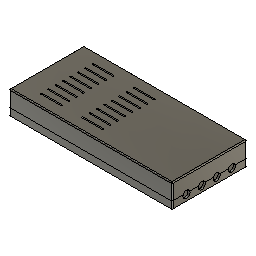
bladeRF_micro_b200_case (Autodesk Fusion 360 design; units mm, degrees)
Autodesk Fusion 360 part; units mm, degrees
(part 1 of 14)
sketch "micro (1)" plane through (0, 0, 0) normal (0, 0, 1) x (1, 0, 0)
  line L0 (35.86, 33.621) -> (35.86, 34.221)
  line L1 (35.86, 34.221) -> (34.76, 34.221)
  line L2 (34.76, 34.221) -> (34.76, 33.621)
  line L3 (41.36, 56.942) -> (41.36, 56.342)
  line L4 (35.818, 34.2258) -> (35.818, 33.6162)
  line L5 (42.46, 59.228) -> (41.36, 59.228)
  line L6 (42.418, 59.2328) -> (42.418, 58.6232)
  line L7 (42.46, 56.942) -> (41.36, 56.942)
  line L8 (35.818, 34.2258) -> (35.818, 33.6162)
  line L9 (42.035, 56.3372) -> (42.035, 56.9468)
  line L10 (41.36, 56.342) -> (42.46, 56.342)
  line L11 (29.591, 15.3162) -> (28.575, 15.3162)
  line L12 (41.785, 58.6232) -> (42.035, 58.6232)
  line L13 (41.785, 56.3372) -> (42.035, 56.3372)
  line L14 (41.402, 56.9468) -> (42.418, 56.9468)
  line L15 (41.402, 58.6232) -> (41.402, 59.2328)
  line L16 (42.035, 58.6232) -> (42.035, 59.2328)
  line L17 (34.76, 33.621) -> (35.86, 33.621)
  line L18 (34.802, 33.6162) -> (34.802, 34.2258)
  line L19 (34.802, 34.2258) -> (35.818, 34.2258)
  line L20 (42.035, 59.2328) -> (41.785, 59.2328)
  line L21 (41.785, 59.2328) -> (41.785, 58.6232)
  line L22 (42.46, 58.628) -> (42.46, 59.228)
  line L23 (41.402, 59.2328) -> (42.418, 59.2328)
  line L24 (35.185, 34.2258) -> (35.185, 33.6162)
  line L25 (35.818, 33.6162) -> (34.802, 33.6162)
  line L26 (35.818, 33.6162) -> (34.802, 33.6162)
  line L27 (42.418, 59.2328) -> (42.418, 58.6232)
  line L28 (42.418, 56.3372) -> (41.402, 56.3372)
  line L29 (29.591, 15.9258) -> (29.591, 15.3162)
  line L30 (41.402, 56.9468) -> (42.418, 56.9468)
  line L31 (42.418, 56.9468) -> (42.418, 56.3372)
  line L32 (41.402, 56.3372) -> (41.402, 56.9468)
  line L33 (21.124, 5.507) -> (20.024, 5.507)
  line L34 (20.024, 5.507) -> (20.024, 4.907)
  line L35 (35.435, 34.2258) -> (35.185, 34.2258)
  line L36 (20.024, 6.65) -> (20.024, 6.05)
  line L37 (29.591, 15.9258) -> (29.591, 15.3162)
  line L38 (41.36, 59.228) -> (41.36, 58.628)
  line L39 (28.958, 15.9258) -> (28.958, 15.3162)
  line L40 (21.082, 6.6548) -> (21.082, 6.0452)
  line L41 (20.066, 4.9022) -> (20.066, 5.5118)
  line L42 (20.449, 4.9022) -> (20.699, 4.9022)
  line L43 (21.082, 5.5118) -> (21.082, 4.9022)
  line L44 (20.066, 4.9022) -> (20.066, 5.5118)
  line L45 (35.185, 33.6162) -> (35.435, 33.6162)
  line L46 (21.124, 6.65) -> (20.024, 6.65)
  line L47 (34.802, 33.6162) -> (34.802, 34.2258)
  line L48 (21.082, 6.0452) -> (20.066, 6.0452)
  line L49 (21.124, 4.907) -> (21.124, 5.507)
  line L50 (6.35, 56.896) -> (6.35, 57.404)
  arc A0 (88.9, 59.69) -> (88.9, 54.61) centre (88.9, 57.15) ccw
  arc A1 (7.9248, 57.15) -> (4.7752, 57.15) centre (6.35, 57.15) ccw
  arc A2 (88.9, 59.69) -> (88.9, 54.61) centre (88.9, 57.15) ccw
  arc A3 (7.9248, 57.15) -> (4.7752, 57.15) centre (6.35, 57.15) ccw
  line L51 (6.096, 57.15) -> (6.604, 57.15)
  line L52 (88.9, 56.896) -> (88.9, 57.404)
  arc A4 (88.9, 54.61) -> (88.9, 59.69) centre (88.9, 57.15) ccw
  arc A5 (88.9, 56.3689) -> (88.9, 57.931) centre (88.9, 57.15) ccw
  arc A6 (88.9, 55.5879) -> (88.9, 58.7121) centre (88.9, 57.15) ccw
  arc A7 (6.35, 56.8007) -> (6.35, 57.4992) centre (6.35, 57.15) ccw
  line L53 (88.646, 57.15) -> (89.154, 57.15)
  arc A8 (6.35, 58.42) -> (6.35, 55.88) centre (6.35, 57.15) ccw
  line L54 (6.096, 57.15) -> (6.604, 57.15)
  arc A9 (6.35, 57.4992) -> (6.35, 56.8007) centre (6.35, 57.15) ccw
  line L55 (6.096, 57.15) -> (6.604, 57.15)
  arc A10 (88.9, 55.88) -> (88.9, 58.42) centre (88.9, 57.15) ccw
  arc A11 (5.7086, 57.15) -> (6.9913, 57.15) centre (6.35, 57.15) ccw
  arc A12 (5.7086, 57.15) -> (6.9913, 57.15) centre (6.35, 57.15) ccw
  line L56 (6.35, 56.896) -> (6.35, 57.404)
  arc A13 (88.9, 54.61) -> (88.9, 59.69) centre (88.9, 57.15) ccw
  arc A14 (6.9913, 57.15) -> (5.7086, 57.15) centre (6.35, 57.15) ccw
  arc A15 (88.9, 56.8007) -> (88.9, 57.4992) centre (88.9, 57.15) ccw
  line L57 (6.096, 57.15) -> (6.604, 57.15)
  arc A16 (6.35, 54.61) -> (6.35, 59.69) centre (6.35, 57.15) ccw
  line L58 (6.096, 57.15) -> (6.604, 57.15)
  arc A17 (5.7086, 57.15) -> (6.9913, 57.15) centre (6.35, 57.15) ccw
  arc A18 (6.9913, 57.15) -> (5.7086, 57.15) centre (6.35, 57.15) ccw
  arc A19 (88.9, 55.5879) -> (88.9, 58.7121) centre (88.9, 57.15) ccw
  arc A20 (6.35, 59.69) -> (6.35, 54.61) centre (6.35, 57.15) ccw
  line L59 (6.35, 56.896) -> (6.35, 57.404)
  arc A21 (6.35, 55.5879) -> (6.35, 58.7121) centre (6.35, 57.15) ccw
  arc A22 (6.35, 58.42) -> (6.35, 55.88) centre (6.35, 57.15) ccw
  arc A23 (5.7086, 57.15) -> (6.9913, 57.15) centre (6.35, 57.15) ccw
  arc A24 (6.35, 55.88) -> (6.35, 58.42) centre (6.35, 57.15) ccw
  arc A25 (6.35, 55.5879) -> (6.35, 58.7121) centre (6.35, 57.15) ccw
  arc A26 (6.35, 59.69) -> (6.35, 54.61) centre (6.35, 57.15) ccw
  arc A27 (5.7086, 57.15) -> (6.9913, 57.15) centre (6.35, 57.15) ccw
  line L60 (6.096, 57.15) -> (6.604, 57.15)
  arc A28 (6.35, 54.61) -> (6.35, 59.69) centre (6.35, 57.15) ccw
  arc A29 (6.35, 55.88) -> (6.35, 58.42) centre (6.35, 57.15) ccw
  arc A30 (7.9248, 6.35) -> (4.7752, 6.35) centre (6.35, 6.35) ccw
  arc A31 (7.9248, 6.35) -> (4.7752, 6.35) centre (6.35, 6.35) ccw
  arc A32 (5.7086, 57.15) -> (6.9913, 57.15) centre (6.35, 57.15) ccw
  arc A33 (6.9913, 57.15) -> (5.7086, 57.15) centre (6.35, 57.15) ccw
  arc A34 (6.35, 59.69) -> (6.35, 54.61) centre (6.35, 57.15) ccw
  arc A35 (4.7752, 6.35) -> (7.9248, 6.35) centre (6.35, 6.35) ccw
  line L61 (6.35, 56.896) -> (6.35, 57.404)
  arc A36 (6.35, 58.7121) -> (6.35, 55.5879) centre (6.35, 57.15) ccw
  arc A37 (4.7752, 6.35) -> (7.9248, 6.35) centre (6.35, 6.35) ccw
  arc A38 (6.9913, 57.15) -> (5.7086, 57.15) centre (6.35, 57.15) ccw
  arc A39 (5.7086, 57.15) -> (6.9913, 57.15) centre (6.35, 57.15) ccw
  line L62 (6.35, 56.896) -> (6.35, 57.404)
  arc A40 (5.7086, 57.15) -> (6.9913, 57.15) centre (6.35, 57.15) ccw
  arc A41 (6.35, 58.42) -> (6.35, 55.88) centre (6.35, 57.15) ccw
  arc A42 (6.35, 58.42) -> (6.35, 55.88) centre (6.35, 57.15) ccw
  arc A43 (6.35, 58.7121) -> (6.35, 55.5879) centre (6.35, 57.15) ccw
  line L63 (6.35, 56.896) -> (6.35, 57.404)
  arc A44 (6.35, 55.88) -> (6.35, 58.42) centre (6.35, 57.15) ccw
  arc A45 (6.9913, 57.15) -> (5.7086, 57.15) centre (6.35, 57.15) ccw
  arc A46 (6.35, 59.69) -> (6.35, 54.61) centre (6.35, 57.15) ccw
  line L64 (6.096, 57.15) -> (6.604, 57.15)
  arc A47 (6.35, 54.61) -> (6.35, 59.69) centre (6.35, 57.15) ccw
  arc A48 (6.35, 56.3689) -> (6.35, 57.931) centre (6.35, 57.15) ccw
  arc A49 (6.35, 54.61) -> (6.35, 59.69) centre (6.35, 57.15) ccw
  arc A50 (6.35, 57.931) -> (6.35, 56.3689) centre (6.35, 57.15) ccw
  arc A51 (6.9913, 6.35) -> (5.7086, 6.35) centre (6.35, 6.35) ccw
  line L65 (6.35, 6.096) -> (6.35, 6.604)
  arc A52 (6.9913, 6.35) -> (5.7086, 6.35) centre (6.35, 6.35) ccw
  arc A53 (6.9913, 57.15) -> (5.7086, 57.15) centre (6.35, 57.15) ccw
  line L66 (6.096, 57.15) -> (6.604, 57.15)
  arc A54 (6.35, 55.88) -> (6.35, 58.42) centre (6.35, 57.15) ccw
  arc A55 (5.7086, 6.35) -> (6.9913, 6.35) centre (6.35, 6.35) ccw
  line L67 (6.096, 6.35) -> (6.604, 6.35)
  line L68 (6.35, 6.096) -> (6.35, 6.604)
  line L69 (6.096, 6.35) -> (6.604, 6.35)
  line L70 (6.096, 6.35) -> (6.604, 6.35)
  line L71 (6.096, 6.35) -> (6.604, 6.35)
  arc A56 (6.9913, 6.35) -> (5.7086, 6.35) centre (6.35, 6.35) ccw
  arc A57 (5.7086, 6.35) -> (6.9913, 6.35) centre (6.35, 6.35) ccw
  arc A58 (6.35, 8.89) -> (6.35, 3.81) centre (6.35, 6.35) ccw
  arc A59 (5.7086, 6.35) -> (6.9913, 6.35) centre (6.35, 6.35) ccw
  line L72 (6.096, 6.35) -> (6.604, 6.35)
  arc A60 (6.9913, 6.35) -> (5.7086, 6.35) centre (6.35, 6.35) ccw
  line L73 (6.35, 56.896) -> (6.35, 57.404)
  arc A61 (6.9913, 6.35) -> (5.7086, 6.35) centre (6.35, 6.35) ccw
  line L74 (6.35, 56.896) -> (6.35, 57.404)
  arc A62 (5.7086, 6.35) -> (6.9913, 6.35) centre (6.35, 6.35) ccw
  arc A63 (5.7086, 6.35) -> (6.9913, 6.35) centre (6.35, 6.35) ccw
  line L75 (6.096, 6.35) -> (6.604, 6.35)
  line L76 (6.35, 6.096) -> (6.35, 6.604)
  arc A64 (5.7086, 6.35) -> (6.9913, 6.35) centre (6.35, 6.35) ccw
  arc A65 (5.7086, 6.35) -> (6.9913, 6.35) centre (6.35, 6.35) ccw
  arc A66 (6.9913, 6.35) -> (5.7086, 6.35) centre (6.35, 6.35) ccw
  arc A67 (6.9913, 6.35) -> (5.7086, 6.35) centre (6.35, 6.35) ccw
  arc A68 (6.35, 3.81) -> (6.35, 8.89) centre (6.35, 6.35) ccw
  line L77 (6.35, 6.096) -> (6.35, 6.604)
  arc A69 (6.9913, 6.35) -> (5.7086, 6.35) centre (6.35, 6.35) ccw
  arc A70 (5.7086, 6.35) -> (6.9913, 6.35) centre (6.35, 6.35) ccw
  line L78 (6.096, 6.35) -> (6.604, 6.35)
  arc A71 (6.9913, 6.35) -> (5.7086, 6.35) centre (6.35, 6.35) ccw
  line L79 (6.35, 6.096) -> (6.35, 6.604)
  line L80 (6.35, 6.096) -> (6.35, 6.604)
  arc A72 (6.35, 5.5689) -> (6.35, 7.131) centre (6.35, 6.35) ccw
  line L81 (6.35, 6.096) -> (6.35, 6.604)
  arc A73 (6.35, 4.7879) -> (6.35, 7.9121) centre (6.35, 6.35) ccw
  arc A74 (5.7086, 6.35) -> (6.9913, 6.35) centre (6.35, 6.35) ccw
  line L82 (29.573, 16.4652) -> (28.557, 16.4652)
  line L83 (6.096, 6.35) -> (6.604, 6.35)
  line L84 (28.557, 21.1388) -> (29.573, 21.1388)
  line L85 (29.19, 17.4812) -> (29.19, 18.0908)
  line L86 (6.096, 6.35) -> (6.604, 6.35)
  arc A75 (6.35, 4.7879) -> (6.35, 7.9121) centre (6.35, 6.35) ccw
  line L87 (28.515, 17.07) -> (28.515, 16.47)
  line L88 (29.615, 16.47) -> (29.615, 17.07)
  line L89 (28.557, 17.0748) -> (29.573, 17.0748)
  arc A76 (6.35, 8.89) -> (6.35, 3.81) centre (6.35, 6.35) ccw
  arc A77 (6.9913, 6.35) -> (5.7086, 6.35) centre (6.35, 6.35) ccw
  arc A78 (6.35, 7.131) -> (6.35, 5.5689) centre (6.35, 6.35) ccw
  line L90 (6.096, 6.35) -> (6.604, 6.35)
  arc A79 (6.35, 7.9121) -> (6.35, 4.7879) centre (6.35, 6.35) ccw
  arc A80 (5.7086, 6.35) -> (6.9913, 6.35) centre (6.35, 6.35) ccw
  arc A81 (6.35, 7.9121) -> (6.35, 4.7879) centre (6.35, 6.35) ccw
  arc A82 (6.35, 3.81) -> (6.35, 8.89) centre (6.35, 6.35) ccw
  line L91 (28.557, 18.0908) -> (29.573, 18.0908)
  line L92 (6.35, 6.096) -> (6.35, 6.604)
  line L93 (29.19, 21.1388) -> (28.94, 21.1388)
  line L94 (29.615, 18.086) -> (28.515, 18.086)
  line L95 (6.35, 6.096) -> (6.35, 6.604)
  line L96 (28.557, 18.0908) -> (29.573, 18.0908)
  line L97 (28.557, 16.4652) -> (28.557, 17.0748)
  line L98 (6.35, 6.096) -> (6.35, 6.604)
  line L99 (28.557, 17.4812) -> (28.557, 18.0908)
  line L100 (29.208, 15.3162) -> (29.208, 15.9258)
  line L101 (28.94, 21.1388) -> (28.94, 20.5292)
  line L102 (28.515, 16.47) -> (29.615, 16.47)
  line L103 (29.573, 18.0908) -> (29.573, 17.4812)
  line L104 (29.573, 21.1388) -> (29.573, 20.5292)
  line L105 (29.573, 17.4812) -> (28.557, 17.4812)
  line L106 (29.573, 16.4652) -> (28.557, 16.4652)
  line L107 (29.19, 16.4652) -> (29.19, 17.0748)
  line L108 (29.573, 18.0908) -> (29.573, 17.4812)
  line L109 (28.94, 20.5292) -> (29.19, 20.5292)
  arc A83 (77.273, 25.0129) -> (77.273, 24.8351) centre (77.273, 24.924) ccw
  line L110 (29.633, 15.921) -> (28.533, 15.921)
  line L111 (29.19, 20.5292) -> (29.19, 21.1388)
  line L112 (28.533, 15.921) -> (28.533, 15.321)
  line L113 (29.573, 20.5292) -> (28.557, 20.5292)
  line L114 (28.575, 15.9258) -> (29.591, 15.9258)
  line L115 (29.573, 17.4812) -> (28.557, 17.4812)
  line L116 (28.533, 15.321) -> (29.633, 15.321)
  line L117 (29.19, 17.0748) -> (28.94, 17.0748)
  line L118 (28.515, 17.486) -> (29.615, 17.486)
  line L119 (28.557, 16.4652) -> (28.557, 17.0748)
  line L120 (28.94, 16.4652) -> (29.19, 16.4652)
  line L121 (28.94, 17.4812) -> (29.19, 17.4812)
  line L122 (29.633, 15.321) -> (29.633, 15.921)
  line L123 (28.515, 18.086) -> (28.515, 17.486)
  line L124 (29.615, 17.07) -> (28.515, 17.07)
  line L125 (29.19, 18.0908) -> (28.94, 18.0908)
  line L126 (28.557, 17.0748) -> (29.573, 17.0748)
  line L127 (28.575, 15.3162) -> (28.575, 15.9258)
  line L128 (29.573, 17.0748) -> (29.573, 16.4652)
  line L129 (28.94, 17.0748) -> (28.94, 16.4652)
  line L130 (29.591, 15.3162) -> (28.575, 15.3162)
  line L131 (28.557, 17.4812) -> (28.557, 18.0908)
  line L132 (41.402, 59.2328) -> (42.418, 59.2328)
  line L133 (28.94, 18.0908) -> (28.94, 17.4812)
  line L134 (29.573, 17.0748) -> (29.573, 16.4652)
  line L135 (29.615, 17.486) -> (29.615, 18.086)
  line L136 (41.36, 58.628) -> (42.46, 58.628)
  line L137 (41.402, 56.3372) -> (41.402, 56.9468)
  line L138 (28.958, 15.3162) -> (29.208, 15.3162)
  line L139 (28.575, 15.3162) -> (28.575, 15.9258)
  line L140 (41.402, 58.6232) -> (41.402, 59.2328)
  line L141 (42.418, 58.6232) -> (41.402, 58.6232)
  line L142 (28.575, 15.9258) -> (29.591, 15.9258)
  line L143 (42.46, 56.342) -> (42.46, 56.942)
  line L144 (42.418, 56.9468) -> (42.418, 56.3372)
  line L145 (42.418, 58.6232) -> (41.402, 58.6232)
  line L146 (42.418, 56.3372) -> (41.402, 56.3372)
  line L147 (42.035, 56.9468) -> (41.785, 56.9468)
  line L148 (41.785, 56.9468) -> (41.785, 56.3372)
  line L149 (29.208, 15.9258) -> (28.958, 15.9258)
  line L150 (29.0068, 38.862) -> (33.5788, 38.862)
  arc A84 (95.042, 49.8688) -> (95.042, 49.8692) centre (95.042, 49.869) ccw
  line L151 (29.083, 46.2788) -> (33.5534, 46.2788)
  arc A85 (95.042, 49.8692) -> (95.042, 49.8688) centre (95.042, 49.869) ccw
  arc A86 (94.442, 49.8692) -> (94.442, 49.8688) centre (94.442, 49.869) ccw
  arc A87 (94.442, 49.8688) -> (94.442, 49.8692) centre (94.442, 49.869) ccw
  line L152 (29.9974, 45.72) -> (32.5882, 45.72)
  line L153 (95.042, 49.869) -> (95.042, 50.969)
  line L154 (29.9974, 45.72) -> (32.5882, 45.72)
  line L155 (94.6912, 5.336) -> (95.3008, 5.336)
  line L156 (95.0468, 50.544) -> (94.4372, 50.544)
  arc A88 (95.042, 50.9692) -> (95.042, 50.9688) centre (95.042, 50.969) ccw
  line L157 (95.3008, 5.969) -> (95.3008, 4.953)
  arc A89 (95.042, 50.9688) -> (95.042, 50.9692) centre (95.042, 50.969) ccw
  line L158 (29.0068, 46.482) -> (29.0068, 38.862)
  line L159 (33.5788, 46.482) -> (29.0068, 46.482)
  line L160 (29.0576, 45.8978) -> (33.5534, 45.8978)
  line L161 (94.6912, 5.586) -> (94.6912, 5.336)
  arc A90 (95.296, 6.0108) -> (95.296, 6.0112) centre (95.296, 6.011) ccw
  line L162 (29.0068, 46.482) -> (29.0068, 38.862)
  line L163 (94.442, 49.869) -> (95.042, 49.869)
  line L164 (95.3008, 4.953) -> (94.6912, 4.953)
  line L165 (33.5788, 38.862) -> (33.5788, 46.482)
  arc A91 (94.442, 50.9688) -> (94.442, 50.9692) centre (94.442, 50.969) ccw
  line L166 (35.435, 40.1948) -> (35.185, 40.1948)
  line L167 (34.76, 40.19) -> (34.76, 39.59)
  line L168 (34.802, 40.1948) -> (35.818, 40.1948)
  line L169 (35.818, 39.5852) -> (34.802, 39.5852)
  line L170 (73.025, 20.3962) -> (73.025, 21.0058)
  line L171 (29.0068, 38.862) -> (33.5788, 38.862)
  arc A92 (35.8597, 40.19) -> (35.8602, 40.19) centre (35.86, 40.19) ccw
  line L172 (95.042, 50.969) -> (94.442, 50.969)
  arc A93 (35.8602, 39.59) -> (35.8597, 39.59) centre (35.86, 39.59) ccw
  line L173 (29.083, 46.0756) -> (29.083, 46.2788)
  line L174 (94.6912, 4.953) -> (94.6912, 5.969)
  arc A94 (72.9828, 21.001) -> (72.9832, 21.001) centre (72.983, 21.001) ccw
  line L175 (73.408, 17.6022) -> (73.658, 17.6022)
  line L176 (74.083, 21.001) -> (72.983, 21.001)
  line L177 (29.9974, 45.72) -> (32.5882, 45.72)
  arc A95 (72.9832, 21.001) -> (72.9828, 21.001) centre (72.983, 21.001) ccw
  line L178 (74.041, 18.2118) -> (74.041, 17.6022)
  arc A96 (74.0828, 21.001) -> (74.0832, 21.001) centre (74.083, 21.001) ccw
  line L179 (33.5534, 45.8978) -> (33.5534, 46.0756)
  arc A97 (95.296, 6.0112) -> (95.296, 6.0108) centre (95.296, 6.011) ccw
  line L180 (33.909, 47.3964) -> (33.0962, 47.3964)
  line L181 (95.296, 4.911) -> (95.296, 6.011)
  line L182 (94.6912, 5.969) -> (95.3008, 5.969)
  line L183 (29.9974, 39.624) -> (32.5882, 39.624)
  line L184 (95.3008, 5.969) -> (95.3008, 4.953)
  line L185 (94.6912, 5.969) -> (95.3008, 5.969)
  line L186 (73.658, 21.0058) -> (73.408, 21.0058)
  line L187 (74.041, 21.0058) -> (74.041, 20.3962)
  line L188 (73.658, 18.2118) -> (73.408, 18.2118)
  line L189 (33.5534, 46.0756) -> (29.083, 46.0756)
  line L190 (29.9974, 39.624) -> (32.5882, 39.624)
  line L191 (33.5788, 38.862) -> (33.5788, 46.482)
  line L192 (95.3008, 5.336) -> (95.3008, 5.586)
  line L193 (33.5026, 47.7774) -> (33.5026, 46.99)
  line L194 (94.6912, 4.953) -> (94.6912, 5.969)
  line L195 (95.3008, 4.953) -> (94.6912, 4.953)
  line L196 (29.9974, 39.624) -> (32.5882, 39.624)
  line L197 (94.442, 50.969) -> (94.442, 49.869)
  line L198 (33.5788, 46.482) -> (29.0068, 46.482)
  arc A98 (94.442, 50.9692) -> (94.442, 50.9688) centre (94.442, 50.969) ccw
  line L199 (21.5392, 24.511) -> (21.5392, 25.527)
  arc A99 (23.16, 25.5692) -> (23.16, 25.5688) centre (23.16, 25.569) ccw
  line L200 (21.5392, 24.894) -> (22.1488, 24.894)
  line L201 (68.411, 32.558) -> (68.411, 31.958)
  line L202 (34.76, 39.59) -> (35.86, 39.59)
  line L203 (69.469, 31.9532) -> (68.453, 31.9532)
  arc A100 (68.4108, 32.558) -> (68.4112, 32.558) centre (68.411, 32.558) ccw
  line L204 (34.802, 39.5852) -> (34.802, 40.1948)
  line L205 (21.544, 25.569) -> (21.544, 24.469)
  arc A101 (22.144, 24.4692) -> (22.144, 24.4688) centre (22.144, 24.469) ccw
  arc A102 (34.7598, 40.19) -> (34.7602, 40.19) centre (34.76, 40.19) ccw
  arc A103 (22.144, 24.4688) -> (22.144, 24.4692) centre (22.144, 24.469) ccw
  line L206 (94.4372, 50.927) -> (95.0468, 50.927)
  line L207 (69.086, 31.9532) -> (69.086, 32.5628)
  line L208 (68.836, 32.5628) -> (68.836, 31.9532)
  arc A104 (34.7598, 39.59) -> (34.7602, 39.59) centre (34.76, 39.59) ccw
  line L209 (22.1488, 24.511) -> (21.5392, 24.511)
  line L210 (23.16, 24.469) -> (23.16, 25.569)
  arc A105 (69.5108, 31.958) -> (69.5112, 31.958) centre (69.511, 31.958) ccw
  line L211 (95.0468, 49.911) -> (94.4372, 49.911)
  arc A106 (69.5112, 31.958) -> (69.5108, 31.958) centre (69.511, 31.958) ccw
  line L212 (68.411, 31.958) -> (69.511, 31.958)
  line L213 (34.802, 40.1948) -> (35.818, 40.1948)
  line L214 (95.0468, 50.294) -> (95.0468, 50.544)
  arc A107 (35.8602, 40.19) -> (35.8597, 40.19) centre (35.86, 40.19) ccw
  line L215 (94.4372, 50.544) -> (94.4372, 50.294)
  line L216 (22.144, 25.569) -> (21.544, 25.569)
  arc A108 (22.56, 24.4688) -> (22.56, 24.4692) centre (22.56, 24.469) ccw
  line L217 (35.818, 40.1948) -> (35.818, 39.5852)
  line L218 (69.511, 32.558) -> (68.411, 32.558)
  arc A109 (69.5108, 32.558) -> (69.5112, 32.558) centre (69.511, 32.558) ccw
  arc A110 (69.5112, 32.558) -> (69.5108, 32.558) centre (69.511, 32.558) ccw
  line L219 (35.435, 39.5852) -> (35.435, 40.1948)
  arc A111 (68.4108, 31.958) -> (68.4112, 31.958) centre (68.411, 31.958) ccw
  line L220 (22.1488, 24.894) -> (22.1488, 25.144)
  line L221 (35.86, 40.19) -> (34.76, 40.19)
  arc A112 (35.8597, 39.59) -> (35.8602, 39.59) centre (35.86, 39.59) ccw
  line L222 (94.4372, 49.911) -> (94.4372, 50.927)
  line L223 (21.544, 24.469) -> (22.144, 24.469)
  line L224 (35.185, 40.1948) -> (35.185, 39.5852)
  arc A113 (68.4112, 31.958) -> (68.4108, 31.958) centre (68.411, 31.958) ccw
  line L225 (94.4372, 50.927) -> (95.0468, 50.927)
  line L226 (35.818, 39.5852) -> (34.802, 39.5852)
  line L227 (95.0468, 50.927) -> (95.0468, 49.911)
  line L228 (35.86, 39.59) -> (35.86, 40.19)
  line L229 (35.818, 40.1948) -> (35.818, 39.5852)
  line L230 (69.086, 32.5628) -> (68.836, 32.5628)
  line L231 (94.4372, 49.911) -> (94.4372, 50.927)
  line L232 (95.0468, 50.927) -> (95.0468, 49.911)
  line L233 (34.802, 39.5852) -> (34.802, 40.1948)
  line L234 (35.185, 39.5852) -> (35.435, 39.5852)
  line L235 (95.0468, 49.911) -> (94.4372, 49.911)
  arc A114 (21.544, 25.5692) -> (21.544, 25.5688) centre (21.544, 25.569) ccw
  arc A115 (22.56, 24.4692) -> (22.56, 24.4688) centre (22.56, 24.469) ccw
  line L236 (94.4372, 50.294) -> (95.0468, 50.294)
  line L237 (69.511, 31.958) -> (69.511, 32.558)
  arc A116 (34.7602, 39.59) -> (34.7598, 39.59) centre (34.76, 39.59) ccw
  line L238 (22.1488, 24.511) -> (21.5392, 24.511)
  line L239 (21.5392, 25.527) -> (22.1488, 25.527)
  line L240 (22.1488, 25.527) -> (22.1488, 24.511)
  arc A117 (68.4112, 32.558) -> (68.4108, 32.558) centre (68.411, 32.558) ccw
  arc A118 (34.7602, 40.19) -> (34.7598, 40.19) centre (34.76, 40.19) ccw
  line L241 (81.2038, 20.193) -> (81.2038, 19.177)
  line L242 (79.583, 20.235) -> (79.583, 19.135)
  line L243 (81.199, 20.235) -> (80.599, 20.235)
  arc A119 (80.599, 20.2352) -> (80.599, 20.2348) centre (80.599, 20.235) ccw
  arc A120 (80.599, 20.2348) -> (80.599, 20.2352) centre (80.599, 20.235) ccw
  line L244 (80.5942, 19.81) -> (80.5942, 19.56)
  line L245 (80.899, 20.36) -> (80.899, 19.81)
  line L246 (80.899, 19.56) -> (80.899, 19.01)
  arc A121 (80.599, 19.1352) -> (80.599, 19.1348) centre (80.599, 19.135) ccw
  arc A122 (79.583, 19.1352) -> (79.583, 19.1348) centre (79.583, 19.135) ccw
  line L247 (42.418, 58.0898) -> (42.418, 57.4802)
  line L248 (80.599, 19.135) -> (81.199, 19.135)
  line L249 (81.2038, 19.81) -> (80.5942, 19.81)
  arc A123 (79.583, 20.2348) -> (79.583, 20.2352) centre (79.583, 20.235) ccw
  arc A124 (42.4598, 58.085) -> (42.4602, 58.085) centre (42.46, 58.085) ccw
  line L250 (80.5942, 20.193) -> (81.2038, 20.193)
  line L251 (80.899, 20.36) -> (80.899, 19.81)
  line L252 (83.862, 25.227) -> (83.862, 25.827)
  arc A125 (81.199, 19.1352) -> (81.199, 19.1348) centre (81.199, 19.135) ccw
  line L253 (80.899, 20.36) -> (80.899, 19.81)
  line L254 (95.3008, 42.797) -> (94.6912, 42.797)
  line L255 (41.235, 57.785) -> (41.785, 57.785)
  line L256 (81.2038, 19.177) -> (80.5942, 19.177)
  line L257 (80.5942, 19.177) -> (80.5942, 20.193)
  arc A126 (81.199, 20.2348) -> (81.199, 20.2352) centre (81.199, 20.235) ccw
  line L258 (81.2038, 19.56) -> (81.2038, 19.81)
  line L259 (95.296, 43.222) -> (94.696, 43.222)
  line L260 (81.199, 19.135) -> (81.199, 20.235)
  arc A127 (82.7618, 25.227) -> (82.7622, 25.227) centre (82.762, 25.227) ccw
  line L261 (42.035, 57.785) -> (42.585, 57.785)
  arc A128 (95.296, 42.1222) -> (95.296, 42.1218) centre (95.296, 42.122) ccw
  line L262 (94.996, 41.997) -> (94.996, 42.547)
  line L263 (94.996, 42.797) -> (94.996, 43.347)
  arc A129 (95.296, 43.2218) -> (95.296, 43.2222) centre (95.296, 43.222) ccw
  line L264 (80.899, 19.56) -> (80.899, 19.01)
  line L265 (94.996, 41.997) -> (94.996, 42.547)
  line L266 (80.599, 20.235) -> (80.599, 19.135)
  line L267 (79.883, 19.56) -> (79.883, 19.01)
  line L268 (94.996, 42.797) -> (94.996, 43.347)
  line L269 (95.296, 42.122) -> (95.296, 43.222)
  line L270 (81.2038, 19.177) -> (80.5942, 19.177)
  line L271 (80.5942, 19.177) -> (80.5942, 20.193)
  line L272 (80.5942, 19.56) -> (81.2038, 19.56)
  arc A130 (80.599, 19.1348) -> (80.599, 19.1352) centre (80.599, 19.135) ccw
  line L273 (80.1878, 19.81) -> (79.5782, 19.81)
  line L274 (41.402, 57.4802) -> (41.402, 58.0898)
  arc A131 (81.199, 20.2352) -> (81.199, 20.2348) centre (81.199, 20.235) ccw
  line L275 (94.996, 41.997) -> (94.996, 42.547)
  arc A132 (95.296, 42.1218) -> (95.296, 42.1222) centre (95.296, 42.122) ccw
  line L276 (94.6912, 42.547) -> (95.3008, 42.547)
  arc A133 (95.296, 43.2222) -> (95.296, 43.2218) centre (95.296, 43.222) ccw
  arc A134 (42.4602, 58.085) -> (42.4598, 58.085) centre (42.46, 58.085) ccw
  line L277 (95.3008, 42.164) -> (94.6912, 42.164)
  line L278 (80.899, 19.56) -> (80.899, 19.01)
  line L279 (94.6912, 42.797) -> (94.6912, 42.547)
  line L280 (95.3008, 42.547) -> (95.3008, 42.797)
  arc A135 (81.199, 19.1348) -> (81.199, 19.1352) centre (81.199, 19.135) ccw
  line L281 (80.5942, 20.193) -> (81.2038, 20.193)
  line L282 (81.2038, 20.193) -> (81.2038, 19.177)
  line L283 (94.996, 42.797) -> (94.996, 43.347)
  line L284 (80.1878, 20.193) -> (80.1878, 19.177)
  arc A136 (80.183, 19.1352) -> (80.183, 19.1348) centre (80.183, 19.135) ccw
  line L285 (82.804, 25.2222) -> (82.804, 25.8318)
  arc A137 (79.583, 20.2352) -> (79.583, 20.2348) centre (79.583, 20.235) ccw
  line L286 (83.187, 24.8158) -> (83.187, 24.2062)
  line L287 (83.862, 24.211) -> (83.862, 24.811)
  line L288 (82.804, 25.8318) -> (83.82, 25.8318)
  arc A138 (82.7622, 25.227) -> (82.7618, 25.227) centre (82.762, 25.227) ccw
  line L289 (80.183, 19.135) -> (80.183, 20.235)
  line L290 (82.804, 24.8158) -> (83.82, 24.8158)
  line L291 (83.82, 25.8318) -> (83.82, 25.2222)
  arc A139 (78.151, 19.2618) -> (78.151, 19.2622) centre (78.151, 19.262) ccw
  line L292 (80.183, 20.235) -> (79.583, 20.235)
  line L293 (79.883, 20.36) -> (79.883, 19.81)
  line L294 (83.82, 25.2222) -> (82.804, 25.2222)
  line L295 (83.862, 25.827) -> (82.762, 25.827)
  line L296 (83.82, 25.8318) -> (83.82, 25.2222)
  arc A140 (82.7622, 25.827) -> (82.7618, 25.827) centre (82.762, 25.827) ccw
  line L297 (83.82, 25.2222) -> (82.804, 25.2222)
  line L298 (82.762, 25.227) -> (83.862, 25.227)
  line L299 (79.5782, 19.56) -> (80.1878, 19.56)
  line L300 (79.5782, 19.177) -> (79.5782, 20.193)
  line L301 (79.5782, 19.177) -> (79.5782, 20.193)
  line L302 (79.883, 20.36) -> (79.883, 19.81)
  line L303 (80.1878, 19.177) -> (79.5782, 19.177)
  line L304 (82.762, 24.811) -> (82.762, 24.211)
  line L305 (83.437, 25.2222) -> (83.437, 25.8318)
  line L306 (82.762, 25.827) -> (82.762, 25.227)
  line L307 (79.883, 19.56) -> (79.883, 19.01)
  arc A141 (83.8622, 25.827) -> (83.8618, 25.827) centre (83.862, 25.827) ccw
  line L308 (77.551, 20.362) -> (77.551, 19.262)
  arc A142 (80.183, 19.1348) -> (80.183, 19.1352) centre (80.183, 19.135) ccw
  line L309 (79.583, 19.135) -> (80.183, 19.135)
  line L310 (79.5782, 19.81) -> (79.5782, 19.56)
  line L311 (83.82, 24.2062) -> (82.804, 24.2062)
  line L312 (82.804, 25.8318) -> (83.82, 25.8318)
  arc A143 (80.183, 20.2352) -> (80.183, 20.2348) centre (80.183, 20.235) ccw
  line L313 (82.804, 25.2222) -> (82.804, 25.8318)
  line L314 (82.637, 25.527) -> (83.187, 25.527)
  arc A144 (79.583, 19.1348) -> (79.583, 19.1352) centre (79.583, 19.135) ccw
  line L315 (79.883, 19.56) -> (79.883, 19.01)
  line L316 (79.883, 20.36) -> (79.883, 19.81)
  line L317 (80.1878, 20.193) -> (80.1878, 19.177)
  line L318 (79.5782, 20.193) -> (80.1878, 20.193)
  line L319 (80.1878, 19.56) -> (80.1878, 19.81)
  line L320 (79.5782, 20.193) -> (80.1878, 20.193)
  line L321 (83.187, 25.8318) -> (83.187, 25.2222)
  arc A145 (83.8622, 24.811) -> (83.8618, 24.811) centre (83.862, 24.811) ccw
  line L322 (80.1878, 19.177) -> (79.5782, 19.177)
  line L323 (77.551, 19.262) -> (78.151, 19.262)
  arc A146 (83.8622, 25.227) -> (83.8618, 25.227) centre (83.862, 25.227) ccw
  arc A147 (83.8618, 25.227) -> (83.8622, 25.227) centre (83.862, 25.227) ccw
  line L324 (83.82, 24.8158) -> (83.82, 24.2062)
  arc A148 (80.183, 20.2348) -> (80.183, 20.2352) centre (80.183, 20.235) ccw
  line L325 (83.82, 24.2062) -> (82.804, 24.2062)
  line L326 (83.187, 25.2222) -> (83.437, 25.2222)
  arc A149 (83.8618, 25.827) -> (83.8622, 25.827) centre (83.862, 25.827) ccw
  arc A150 (82.7618, 25.827) -> (82.7622, 25.827) centre (82.762, 25.827) ccw
  line L327 (82.637, 25.527) -> (83.187, 25.527)
  arc A151 (82.7622, 24.211) -> (82.7618, 24.211) centre (82.762, 24.211) ccw
  arc A152 (83.8618, 24.811) -> (83.8622, 24.811) centre (83.862, 24.811) ccw
  arc A153 (83.8618, 24.211) -> (83.8622, 24.211) centre (83.862, 24.211) ccw
  arc A154 (77.551, 19.2618) -> (77.551, 19.2622) centre (77.551, 19.262) ccw
  line L328 (82.804, 24.8158) -> (83.82, 24.8158)
  line L329 (82.804, 24.2062) -> (82.804, 24.8158)
  arc A155 (78.151, 20.3618) -> (78.151, 20.3622) centre (78.151, 20.362) ccw
  line L330 (77.5462, 20.32) -> (78.1558, 20.32)
  arc A156 (82.7618, 24.211) -> (82.7622, 24.211) centre (82.762, 24.211) ccw
  arc A157 (77.551, 19.2622) -> (77.551, 19.2618) centre (77.551, 19.262) ccw
  line L331 (78.151, 19.262) -> (78.151, 20.362)
  line L332 (83.437, 25.8318) -> (83.187, 25.8318)
  line L333 (78.1558, 19.304) -> (77.5462, 19.304)
  arc A158 (77.551, 20.3622) -> (77.551, 20.3618) centre (77.551, 20.362) ccw
  line L334 (83.82, 24.8158) -> (83.82, 24.2062)
  line L335 (78.151, 20.362) -> (77.551, 20.362)
  line L336 (77.5462, 19.304) -> (77.5462, 20.32)
  line L337 (83.187, 24.2062) -> (83.437, 24.2062)
  line L338 (78.1558, 19.937) -> (77.5462, 19.937)
  arc A159 (77.551, 20.3618) -> (77.551, 20.3622) centre (77.551, 20.362) ccw
  line L339 (82.804, 24.2062) -> (82.804, 24.8158)
  line L340 (83.437, 24.8158) -> (83.187, 24.8158)
  arc A160 (82.7622, 24.811) -> (82.7618, 24.811) centre (82.762, 24.811) ccw
  arc A161 (82.7618, 24.811) -> (82.7622, 24.811) centre (82.762, 24.811) ccw
  arc A162 (83.8622, 24.211) -> (83.8618, 24.211) centre (83.862, 24.211) ccw
  line L341 (83.862, 24.811) -> (82.762, 24.811)
  line L342 (83.437, 24.2062) -> (83.437, 24.8158)
  arc A163 (78.151, 20.3622) -> (78.151, 20.3618) centre (78.151, 20.362) ccw
  line L343 (75.484, 19.262) -> (75.484, 20.362)
  line L344 (74.083, 18.207) -> (72.983, 18.207)
  line L345 (78.1558, 20.32) -> (78.1558, 19.304)
  arc A164 (75.484, 20.3618) -> (75.484, 20.3622) centre (75.484, 20.362) ccw
  line L346 (74.8792, 19.937) -> (74.8792, 19.687)
  line L347 (73.658, 17.6022) -> (73.658, 18.2118)
  line L348 (74.8792, 19.304) -> (74.8792, 20.32)
  arc A165 (78.151, 19.2622) -> (78.151, 19.2618) centre (78.151, 19.262) ccw
  line L349 (77.5462, 20.32) -> (78.1558, 20.32)
  line L350 (82.637, 25.527) -> (83.187, 25.527)
  line L351 (82.762, 24.211) -> (83.862, 24.211)
  line L352 (74.884, 19.262) -> (75.484, 19.262)
  arc A166 (75.484, 19.2618) -> (75.484, 19.2622) centre (75.484, 19.262) ccw
  arc A167 (74.884, 20.3622) -> (74.884, 20.3618) centre (74.884, 20.362) ccw
  line L353 (74.083, 17.607) -> (74.083, 18.207)
  line L354 (75.4888, 19.304) -> (74.8792, 19.304)
  arc A168 (72.9828, 17.607) -> (72.9832, 17.607) centre (72.983, 17.607) ccw
  arc A169 (74.884, 19.2622) -> (74.884, 19.2618) centre (74.884, 19.262) ccw
  line L355 (77.5462, 19.304) -> (77.5462, 20.32)
  arc A170 (74.0828, 18.207) -> (74.0832, 18.207) centre (74.083, 18.207) ccw
  arc A171 (72.9832, 18.207) -> (72.9828, 18.207) centre (72.983, 18.207) ccw
  arc A172 (72.9828, 18.207) -> (72.9832, 18.207) centre (72.983, 18.207) ccw
  line L356 (72.983, 17.607) -> (74.083, 17.607)
  arc A173 (72.9832, 17.607) -> (72.9828, 17.607) centre (72.983, 17.607) ccw
  arc A174 (75.484, 20.3622) -> (75.484, 20.3618) centre (75.484, 20.362) ccw
  arc A175 (74.884, 20.3618) -> (74.884, 20.3622) centre (74.884, 20.362) ccw
  line L357 (75.4888, 20.32) -> (75.4888, 19.304)
  line L358 (75.4888, 19.937) -> (74.8792, 19.937)
  line L359 (74.8792, 19.304) -> (74.8792, 20.32)
  line L360 (73.025, 17.6022) -> (73.025, 18.2118)
  line L361 (74.8792, 20.32) -> (75.4888, 20.32)
  line L362 (77.5462, 19.687) -> (78.1558, 19.687)
  line L363 (75.4888, 19.304) -> (74.8792, 19.304)
  line L364 (78.1558, 20.32) -> (78.1558, 19.304)
  arc A176 (74.0832, 18.207) -> (74.0828, 18.207) centre (74.083, 18.207) ccw
  line L365 (74.884, 20.362) -> (74.884, 19.262)
  line L366 (78.1558, 19.687) -> (78.1558, 19.937)
  arc A177 (74.0832, 17.607) -> (74.0828, 17.607) centre (74.083, 17.607) ccw
  line L367 (78.1558, 19.304) -> (77.5462, 19.304)
  line L368 (75.4888, 19.687) -> (75.4888, 19.937)
  line L369 (74.8792, 20.32) -> (75.4888, 20.32)
  line L370 (73.025, 18.2118) -> (74.041, 18.2118)
  arc A178 (75.484, 19.2622) -> (75.484, 19.2618) centre (75.484, 19.262) ccw
  line L371 (73.408, 18.2118) -> (73.408, 17.6022)
  line L372 (75.484, 20.362) -> (74.884, 20.362)
  line L373 (72.983, 18.207) -> (72.983, 17.607)
  arc A179 (74.884, 19.2618) -> (74.884, 19.2622) centre (74.884, 19.262) ccw
  arc A180 (74.0828, 17.607) -> (74.0832, 17.607) centre (74.083, 17.607) ccw
  line L374 (74.041, 18.2118) -> (74.041, 17.6022)
  line L375 (75.4888, 20.32) -> (75.4888, 19.304)
  line L376 (74.8792, 19.687) -> (75.4888, 19.687)
  line L377 (77.5462, 19.937) -> (77.5462, 19.687)
  line L378 (74.041, 20.3962) -> (73.025, 20.3962)
  line L379 (74.041, 20.3962) -> (73.025, 20.3962)
  line L380 (73.408, 20.3962) -> (73.658, 20.3962)
  line L381 (72.983, 21.001) -> (72.983, 20.401)
  arc A181 (94.696, 4.9112) -> (94.696, 4.9108) centre (94.696, 4.911) ccw
  arc A182 (94.696, 6.0112) -> (94.696, 6.0108) centre (94.696, 6.011) ccw
  line L382 (94.696, 4.911) -> (95.296, 4.911)
  line L383 (74.041, 21.0058) -> (74.041, 20.3962)
  line L384 (72.983, 20.401) -> (74.083, 20.401)
  line L385 (74.041, 17.6022) -> (73.025, 17.6022)
  line L386 (73.025, 17.6022) -> (73.025, 18.2118)
  line L387 (73.025, 20.3962) -> (73.025, 21.0058)
  arc A183 (74.0832, 21.001) -> (74.0828, 21.001) centre (74.083, 21.001) ccw
  line L388 (73.025, 21.0058) -> (74.041, 21.0058)
  arc A184 (95.296, 4.9108) -> (95.296, 4.9112) centre (95.296, 4.911) ccw
  arc A185 (74.0832, 20.401) -> (74.0828, 20.401) centre (74.083, 20.401) ccw
  arc A186 (95.296, 4.9112) -> (95.296, 4.9108) centre (95.296, 4.911) ccw
  arc A187 (72.9828, 20.401) -> (72.9832, 20.401) centre (72.983, 20.401) ccw
  line L389 (94.696, 6.011) -> (94.696, 4.911)
  line L390 (73.025, 18.2118) -> (74.041, 18.2118)
  line L391 (73.408, 21.0058) -> (73.408, 20.3962)
  line L392 (73.025, 21.0058) -> (74.041, 21.0058)
  arc A188 (94.696, 6.0108) -> (94.696, 6.0112) centre (94.696, 6.011) ccw
  arc A189 (72.9832, 20.401) -> (72.9828, 20.401) centre (72.983, 20.401) ccw
  arc A190 (94.696, 4.9108) -> (94.696, 4.9112) centre (94.696, 4.911) ccw
  arc A191 (74.0828, 20.401) -> (74.0832, 20.401) centre (74.083, 20.401) ccw
  line L393 (74.083, 20.401) -> (74.083, 21.001)
  line L394 (95.296, 6.011) -> (94.696, 6.011)
  line L395 (74.041, 17.6022) -> (73.025, 17.6022)
  line L396 (95.3008, 5.586) -> (94.6912, 5.586)
  line L397 (73.658, 20.3962) -> (73.658, 21.0058)
  arc A192 (83.081, 27.1132) -> (83.081, 27.1767) centre (83.081, 27.145) ccw
  arc A193 (68.73, 21.7183) -> (68.73, 21.7818) centre (68.73, 21.75) ccw
  line L398 (68.7578, 21.8948) -> (68.7578, 22.5552)
  line L399 (16.405, 12.999) -> (15.055, 12.999)
  line L400 (68.4022, 21.8948) -> (68.7578, 21.8948)
  line L401 (68.43, 22.7) -> (68.43, 21.75)
  line L402 (68.73, 22.7) -> (68.43, 22.7)
  line L403 (82.781, 26.195) -> (83.081, 26.195)
  line L404 (68.4022, 22.5552) -> (68.4022, 21.8948)
  arc A194 (68.43, 21.7183) -> (68.43, 21.7818) centre (68.43, 21.75) ccw
  line L405 (83.081, 27.145) -> (82.781, 27.145)
  line L406 (83.081, 26.195) -> (83.081, 27.145)
  line L407 (68.745, 21.91) -> (68.745, 22.54)
  line L408 (68.4022, 22.5552) -> (68.4022, 21.8948)
  line L409 (83.096, 26.355) -> (83.096, 26.985)
  line L410 (68.58, 21.75) -> (68.58, 22.1)
  arc A195 (68.43, 22.6682) -> (68.43, 22.7317) centre (68.43, 22.7) ccw
  line L411 (82.7532, 26.3398) -> (83.1088, 26.3398)
  line L412 (68.7578, 22.5552) -> (68.4022, 22.5552)
  line L413 (68.415, 21.91) -> (68.745, 21.91)
  arc A196 (82.781, 26.1633) -> (82.781, 26.2268) centre (82.781, 26.195) ccw
  line L414 (68.4022, 21.8948) -> (68.7578, 21.8948)
  line L415 (82.7532, 27.0002) -> (82.7532, 26.3398)
  arc A197 (83.081, 26.1633) -> (83.081, 26.2268) centre (83.081, 26.195) ccw
  line L416 (82.931, 27.145) -> (82.931, 26.795)
  line L417 (68.58, 21.75) -> (68.58, 22.1)
  line L418 (68.7578, 21.8948) -> (68.7578, 22.5552)
  line L419 (68.415, 22.54) -> (68.415, 21.91)
  line L420 (16.405, 12.999) -> (15.055, 12.999)
  arc A198 (68.73, 21.7818) -> (68.73, 21.7183) centre (68.73, 21.75) ccw
  arc A199 (68.73, 22.7317) -> (68.73, 22.6682) centre (68.73, 22.7) ccw
  line L421 (16.405, 14.699) -> (15.055, 14.699)
  line L422 (82.781, 27.145) -> (82.781, 26.195)
  arc A200 (68.73, 22.6682) -> (68.73, 22.7317) centre (68.73, 22.7) ccw
  arc A201 (68.43, 21.7818) -> (68.43, 21.7183) centre (68.43, 21.75) ccw
  line L423 (68.58, 21.75) -> (68.58, 22.1)
  line L424 (15.9332, 22.993) -> (14.5108, 22.993)
  line L425 (82.931, 26.545) -> (82.931, 26.195)
  line L426 (83.1088, 27.0002) -> (82.7532, 27.0002)
  line L427 (82.7532, 27.0002) -> (82.7532, 26.3398)
  line L428 (14.5108, 22.993) -> (14.5108, 20.707)
  line L429 (83.1088, 26.3398) -> (83.1088, 27.0002)
  line L430 (14.547, 21) -> (15.897, 21)
  line L431 (83.1088, 26.3398) -> (83.1088, 27.0002)
  line L432 (14.547, 21) -> (15.897, 21)
  line L433 (15.9332, 20.707) -> (15.9332, 22.993)
  line L434 (82.931, 27.145) -> (82.931, 26.795)
  line L435 (82.931, 26.545) -> (82.931, 26.195)
  line L436 (15.9332, 20.707) -> (15.9332, 22.993)
  line L437 (82.766, 26.355) -> (83.096, 26.355)
  line L438 (14.547, 22.7) -> (15.897, 22.7)
  arc A202 (82.781, 27.1132) -> (82.781, 27.1767) centre (82.781, 27.145) ccw
  line L439 (15.9332, 22.993) -> (14.5108, 22.993)
  line L440 (82.931, 27.145) -> (82.931, 26.795)
  line L441 (14.5108, 22.993) -> (14.5108, 20.707)
  arc A203 (83.081, 26.2268) -> (83.081, 26.1633) centre (83.081, 26.195) ccw
  line L442 (14.547, 22.7) -> (15.897, 22.7)
  line L443 (15.947, 20.75) -> (15.947, 22.95)
  line L444 (14.497, 22.95) -> (14.497, 20.75)
  arc A204 (82.781, 26.2268) -> (82.781, 26.1633) centre (82.781, 26.195) ccw
  line L445 (82.931, 26.545) -> (82.931, 26.195)
  line L446 (15.947, 22.95) -> (14.497, 22.95)
  line L447 (83.096, 26.985) -> (82.766, 26.985)
  line L448 (82.766, 26.985) -> (82.766, 26.355)
  line L449 (82.7532, 26.3398) -> (83.1088, 26.3398)
  line L450 (14.5108, 20.707) -> (15.9332, 20.707)
  line L451 (14.547, 21) -> (15.897, 21)
  line L452 (14.547, 22.7) -> (15.897, 22.7)
  line L453 (68.411, 23.668) -> (68.411, 23.068)
  line L454 (14.497, 20.75) -> (15.947, 20.75)
  line L455 (68.411, 23.068) -> (69.511, 23.068)
  line L456 (69.086, 23.0632) -> (69.086, 23.6728)
  line L457 (69.511, 23.668) -> (68.411, 23.668)
  arc A205 (24.389, 25.2778) -> (24.389, 25.2143) centre (24.389, 25.246) ccw
  line L458 (24.239, 24.896) -> (24.239, 25.246)
  line L459 (24.0612, 25.1012) -> (24.0612, 24.4408)
  line L460 (24.4168, 24.4408) -> (24.4168, 25.1012)
  line L461 (25.428, 24.348) -> (25.428, 25.448)
  arc A206 (24.089, 24.2643) -> (24.089, 24.3278) centre (24.089, 24.296) ccw
  line L462 (25.428, 25.448) -> (24.828, 25.448)
  line L463 (68.836, 23.0632) -> (69.086, 23.0632)
  line L464 (69.469, 23.6728) -> (69.469, 23.0632)
  arc A207 (24.089, 25.2143) -> (24.089, 25.2778) centre (24.089, 25.246) ccw
  arc A208 (24.389, 24.3278) -> (24.389, 24.2643) centre (24.389, 24.296) ccw
  line L465 (24.8232, 24.773) -> (25.4328, 24.773)
  line L466 (24.8232, 25.406) -> (25.4328, 25.406)
  line L467 (24.404, 25.086) -> (24.074, 25.086)
  line L468 (68.453, 23.6728) -> (69.469, 23.6728)
  line L469 (24.239, 24.296) -> (24.239, 24.646)
  line L470 (24.239, 24.896) -> (24.239, 25.246)
  line L471 (24.239, 24.896) -> (24.239, 25.246)
  line L472 (24.4168, 25.1012) -> (24.0612, 25.1012)
  line L473 (68.836, 23.6728) -> (68.836, 23.0632)
  line L474 (24.239, 24.296) -> (24.239, 24.646)
  arc A209 (24.089, 24.3278) -> (24.089, 24.2643) centre (24.089, 24.296) ccw
  line L475 (25.4328, 24.39) -> (24.8232, 24.39)
  line L476 (24.089, 25.246) -> (24.089, 24.296)
  line L477 (24.828, 24.348) -> (25.428, 24.348)
  line L478 (69.086, 23.6728) -> (68.836, 23.6728)
  line L479 (24.389, 24.296) -> (24.389, 25.246)
  line L480 (24.0612, 24.4408) -> (24.4168, 24.4408)
  line L481 (84.5019, 26.7033) -> (84.5019, 26.1033)
  line L482 (24.4168, 24.4408) -> (24.4168, 25.1012)
  line L483 (75.8952, 53.848) -> (75.8952, 54.864)
  line L484 (24.828, 25.448) -> (24.828, 24.348)
  line L485 (68.453, 23.0632) -> (68.453, 23.6728)
  line L486 (14.5108, 20.707) -> (15.9332, 20.707)
  arc A210 (24.389, 24.2643) -> (24.389, 24.3278) centre (24.389, 24.296) ccw
  line L487 (24.074, 25.086) -> (24.074, 24.456)
  line L488 (69.469, 23.0632) -> (68.453, 23.0632)
  line L489 (68.453, 23.0632) -> (68.453, 23.6728)
  line L490 (69.511, 23.068) -> (69.511, 23.668)
  line L491 (24.0612, 25.1012) -> (24.0612, 24.4408)
  arc A211 (24.089, 25.2778) -> (24.089, 25.2143) centre (24.089, 25.246) ccw
  line L492 (24.0612, 24.4408) -> (24.4168, 24.4408)
  line L493 (68.453, 23.6728) -> (69.469, 23.6728)
  line L494 (24.389, 25.246) -> (24.089, 25.246)
  line L495 (24.089, 24.296) -> (24.389, 24.296)
  line L496 (25.4328, 25.406) -> (25.4328, 24.39)
  line L497 (24.404, 24.456) -> (24.404, 25.086)
  line L498 (83.1088, 27.0002) -> (82.7532, 27.0002)
  line L499 (69.469, 23.0632) -> (68.453, 23.0632)
  line L500 (24.4168, 25.1012) -> (24.0612, 25.1012)
  line L501 (69.469, 23.6728) -> (69.469, 23.0632)
  arc A212 (24.389, 25.2143) -> (24.389, 25.2778) centre (24.389, 25.246) ccw
  line L502 (24.239, 24.296) -> (24.239, 24.646)
  line L503 (24.074, 24.456) -> (24.404, 24.456)
  line L504 (85.5599, 26.7081) -> (85.5599, 26.0985)
  line L505 (84.5439, 26.7081) -> (85.5599, 26.7081)
  line L506 (85.6019, 26.7033) -> (84.5019, 26.7033)
  line L507 (84.5439, 26.7081) -> (85.5599, 26.7081)
  line L508 (24.8232, 24.39) -> (24.8232, 25.406)
  line L509 (72.7202, 52.324) -> (73.3298, 52.324)
  line L510 (80.052, 58.339) -> (78.952, 58.339)
  line L511 (73.3298, 51.941) -> (72.7202, 51.941)
  line L512 (73.364, 54.656) -> (73.364, 54.056)
  line L513 (75.8952, 54.864) -> (76.5048, 54.864)
  line L514 (84.5439, 26.0985) -> (84.5439, 26.7081)
  line L515 (85.1769, 26.7081) -> (84.9269, 26.7081)
  line L516 (85.5599, 26.0985) -> (84.5439, 26.0985)
  line L517 (78.994, 57.7342) -> (78.994, 58.3438)
  line L518 (24.8232, 25.023) -> (24.8232, 24.773)
  line L519 (75.8952, 54.864) -> (76.5048, 54.864)
  line L520 (78.994, 57.7342) -> (78.994, 58.3438)
  line L521 (79.627, 57.7342) -> (79.627, 58.3438)
  line L522 (80.01, 58.3438) -> (80.01, 57.7342)
  line L523 (78.994, 58.3438) -> (80.01, 58.3438)
  line L524 (85.5599, 26.0985) -> (84.5439, 26.0985)
  line L525 (84.5019, 26.1033) -> (85.6019, 26.1033)
  line L526 (76.5048, 54.864) -> (76.5048, 53.848)
  line L527 (75.9, 54.906) -> (75.9, 53.806)
  line L528 (75.8952, 54.481) -> (75.8952, 54.231)
  line L529 (76.5048, 54.481) -> (75.8952, 54.481)
  line L530 (25.4328, 24.773) -> (25.4328, 25.023)
  line L531 (76.5048, 54.864) -> (76.5048, 53.848)
  line L532 (75.9, 53.806) -> (76.5, 53.806)
  line L533 (78.952, 57.739) -> (80.052, 57.739)
  line L534 (75.8952, 54.231) -> (76.5048, 54.231)
  line L535 (76.5, 54.906) -> (75.9, 54.906)
  line L536 (80.01, 57.7342) -> (78.994, 57.7342)
  line L537 (25.4328, 25.406) -> (25.4328, 24.39)
  line L538 (76.5048, 53.848) -> (75.8952, 53.848)
  line L539 (25.4328, 24.39) -> (24.8232, 24.39)
  line L540 (85.6019, 26.1033) -> (85.6019, 26.7033)
  line L541 (78.952, 58.339) -> (78.952, 57.739)
  line L542 (75.8952, 53.848) -> (75.8952, 54.864)
  line L543 (76.5, 53.806) -> (76.5, 54.906)
  line L544 (78.994, 58.3438) -> (80.01, 58.3438)
  line L545 (85.1769, 26.0985) -> (85.1769, 26.7081)
  line L546 (85.5599, 26.7081) -> (85.5599, 26.0985)
  line L547 (24.8232, 24.39) -> (24.8232, 25.406)
  line L548 (25.4328, 25.023) -> (24.8232, 25.023)
  line L549 (84.9269, 26.7081) -> (84.9269, 26.0985)
  line L550 (80.052, 57.739) -> (80.052, 58.339)
  line L551 (76.5048, 54.231) -> (76.5048, 54.481)
  line L552 (84.5439, 26.0985) -> (84.5439, 26.7081)
  line L553 (76.5048, 53.848) -> (75.8952, 53.848)
  line L554 (24.8232, 25.406) -> (25.4328, 25.406)
  line L555 (80.01, 58.3438) -> (80.01, 57.7342)
  line L556 (84.9269, 26.0985) -> (85.1769, 26.0985)
  line L557 (80.01, 57.7342) -> (78.994, 57.7342)
  line L558 (72.686, 56.307) -> (71.586, 56.307)
  line L559 (72.644, 56.3118) -> (72.644, 55.7022)
  line L560 (72.644, 55.7022) -> (71.628, 55.7022)
  line L561 (74.039, 54.0512) -> (74.039, 54.6608)
  line L562 (72.7202, 51.308) -> (72.7202, 52.324)
  line L563 (72.7202, 52.324) -> (73.3298, 52.324)
  line L564 (73.325, 51.266) -> (73.325, 52.366)
  line L565 (73.406, 54.6608) -> (74.422, 54.6608)
  line L566 (79.377, 57.7342) -> (79.627, 57.7342)
  line L567 (74.422, 54.6608) -> (74.422, 54.0512)
  line L568 (71.628, 56.3118) -> (72.644, 56.3118)
  line L569 (79.627, 58.3438) -> (79.377, 58.3438)
  line L570 (72.7202, 51.941) -> (72.7202, 51.691)
  line L571 (74.422, 54.0512) -> (73.406, 54.0512)
  line L572 (72.686, 55.707) -> (72.686, 56.307)
  line L573 (72.011, 56.3118) -> (72.011, 55.7022)
  line L574 (73.789, 54.6608) -> (73.789, 54.0512)
  line L575 (71.628, 55.7022) -> (71.628, 56.3118)
  line L576 (79.377, 58.3438) -> (79.377, 57.7342)
  line L577 (71.628, 56.3118) -> (72.644, 56.3118)
  line L578 (73.325, 52.366) -> (72.725, 52.366)
  line L579 (72.725, 51.266) -> (73.325, 51.266)
  line L580 (72.261, 55.7022) -> (72.261, 56.3118)
  line L581 (72.7202, 51.691) -> (73.3298, 51.691)
  line L582 (73.3298, 52.324) -> (73.3298, 51.308)
  line L583 (73.364, 54.056) -> (74.464, 54.056)
  line L584 (73.406, 54.0512) -> (73.406, 54.6608)
  line L585 (74.039, 54.6608) -> (73.789, 54.6608)
  line L586 (72.644, 55.7022) -> (71.628, 55.7022)
  line L587 (73.3298, 51.308) -> (72.7202, 51.308)
  line L588 (71.586, 56.307) -> (71.586, 55.707)
  line L589 (73.406, 54.0512) -> (73.406, 54.6608)
  line L590 (73.3298, 51.691) -> (73.3298, 51.941)
  line L591 (74.422, 54.0512) -> (73.406, 54.0512)
  line L592 (72.7202, 51.308) -> (72.7202, 52.324)
  line L593 (70.866, 57.4548) -> (70.866, 56.8452)
  line L594 (70.233, 56.8452) -> (70.483, 56.8452)
  arc A213 (3.048, 3.175) -> (3.048, 2.667) centre (3.048, 2.921) ccw
  line L595 (73.3298, 51.308) -> (72.7202, 51.308)
  line L596 (70.866, 56.8452) -> (69.85, 56.8452)
  arc A214 (92.31, 12.652) -> (92.31, 13.668) centre (92.31, 13.16) ccw
  line L597 (70.866, 56.8452) -> (69.85, 56.8452)
  line L598 (70.866, 57.4548) -> (70.866, 56.8452)
  line L599 (72.011, 55.7022) -> (72.261, 55.7022)
  line L600 (73.789, 54.0512) -> (74.039, 54.0512)
  line L601 (72.725, 52.366) -> (72.725, 51.266)
  line L602 (71.628, 55.7022) -> (71.628, 56.3118)
  line L603 (73.3298, 52.324) -> (73.3298, 51.308)
  line L604 (73.406, 54.6608) -> (74.422, 54.6608)
  line L605 (72.644, 56.3118) -> (72.644, 55.7022)
  line L606 (71.586, 55.707) -> (72.686, 55.707)
  line L607 (74.464, 54.656) -> (73.364, 54.656)
  line L608 (74.422, 54.6608) -> (74.422, 54.0512)
  line L609 (72.261, 56.3118) -> (72.011, 56.3118)
  line L610 (74.464, 54.056) -> (74.464, 54.656)
  arc A215 (9.652, 44.577) -> (9.652, 44.069) centre (9.652, 44.323) ccw
  line L611 (70.908, 56.85) -> (70.908, 57.45)
  line L612 (70.483, 56.8452) -> (70.483, 57.4548)
  arc A216 (10.4245, 44.323) -> (8.8795, 44.323) centre (9.652, 44.323) ccw
  arc A217 (9.652, 44.069) -> (9.652, 44.577) centre (9.652, 44.323) ccw
  arc A218 (3.048, 2.413) -> (3.048, 3.429) centre (3.048, 2.921) ccw
  arc A219 (93.4025, 13.16) -> (91.2175, 13.16) centre (92.31, 13.16) ccw
  line L613 (69.808, 56.85) -> (70.908, 56.85)
  arc A220 (93.0825, 13.16) -> (91.5375, 13.16) centre (92.31, 13.16) ccw
  arc A221 (91.2175, 13.16) -> (93.4025, 13.16) centre (92.31, 13.16) ccw
  arc A222 (4.1405, 2.921) -> (1.9555, 2.921) centre (3.048, 2.921) ccw
  arc A223 (9.652, 44.831) -> (9.652, 43.815) centre (9.652, 44.323) ccw
  arc A224 (10.7445, 44.323) -> (8.5595, 44.323) centre (9.652, 44.323) ccw
  arc A225 (9.652, 44.069) -> (9.652, 44.577) centre (9.652, 44.323) ccw
  line L614 (70.483, 57.4548) -> (70.233, 57.4548)
  arc A226 (91.5375, 13.16) -> (93.0825, 13.16) centre (92.31, 13.16) ccw
  arc A227 (3.048, 2.667) -> (3.048, 3.175) centre (3.048, 2.921) ccw
  arc A228 (8.8795, 44.323) -> (10.4245, 44.323) centre (9.652, 44.323) ccw
  line L615 (69.85, 57.4548) -> (70.866, 57.4548)
  arc A229 (3.048, 3.429) -> (3.048, 2.413) centre (3.048, 2.921) ccw
  arc A230 (2.2755, 2.921) -> (3.8205, 2.921) centre (3.048, 2.921) ccw
  line L616 (69.808, 57.45) -> (69.808, 56.85)
  arc A231 (8.5595, 44.323) -> (10.7445, 44.323) centre (9.652, 44.323) ccw
  line L617 (70.233, 57.4548) -> (70.233, 56.8452)
  arc A232 (88.2587, 6.35) -> (89.5414, 6.35) centre (88.9, 6.35) ccw
  arc A233 (9.652, 43.815) -> (9.652, 44.831) centre (9.652, 44.323) ccw
  arc A234 (88.2587, 6.35) -> (89.5414, 6.35) centre (88.9, 6.35) ccw
  line L618 (88.9, 6.096) -> (88.9, 6.604)
  arc A235 (89.5414, 6.35) -> (88.2587, 6.35) centre (88.9, 6.35) ccw
  arc A236 (88.9, 5.5689) -> (88.9, 7.131) centre (88.9, 6.35) ccw
  arc A237 (89.5414, 6.35) -> (88.2587, 6.35) centre (88.9, 6.35) ccw
  arc A238 (88.2587, 6.35) -> (89.5414, 6.35) centre (88.9, 6.35) ccw
  arc A239 (3.8205, 2.921) -> (2.2755, 2.921) centre (3.048, 2.921) ccw
  arc A240 (88.9, 3.81) -> (88.9, 8.89) centre (88.9, 6.35) ccw
  arc A241 (88.2587, 6.35) -> (89.5414, 6.35) centre (88.9, 6.35) ccw
  arc A242 (88.9, 7.131) -> (88.9, 5.5689) centre (88.9, 6.35) ccw
  arc A243 (90.4748, 6.35) -> (87.3252, 6.35) centre (88.9, 6.35) ccw
  line L619 (88.9, 6.096) -> (88.9, 6.604)
  line L620 (88.646, 6.35) -> (89.154, 6.35)
  arc A244 (9.652, 44.577) -> (9.652, 44.069) centre (9.652, 44.323) ccw
  arc A245 (88.2587, 6.35) -> (89.5414, 6.35) centre (88.9, 6.35) ccw
  arc A246 (92.31, 13.414) -> (92.31, 12.906) centre (92.31, 13.16) ccw
  arc A247 (3.048, 2.667) -> (3.048, 3.175) centre (3.048, 2.921) ccw
  line L621 (88.9, 6.096) -> (88.9, 6.604)
  line L622 (88.9, 6.096) -> (88.9, 6.604)
  arc A248 (92.31, 12.906) -> (92.31, 13.414) centre (92.31, 13.16) ccw
  arc A249 (3.048, 3.175) -> (3.048, 2.667) centre (3.048, 2.921) ccw
  arc A250 (1.9555, 2.921) -> (4.1405, 2.921) centre (3.048, 2.921) ccw
  line L623 (70.908, 57.45) -> (69.808, 57.45)
  line L624 (69.85, 56.8452) -> (69.85, 57.4548)
  line L625 (69.85, 57.4548) -> (70.866, 57.4548)
  line L626 (69.85, 56.8452) -> (69.85, 57.4548)
  arc A251 (88.2587, 57.15) -> (89.5414, 57.15) centre (88.9, 57.15) ccw
  arc A252 (89.5414, 6.35) -> (88.2587, 6.35) centre (88.9, 6.35) ccw
  arc A253 (88.9, 3.81) -> (88.9, 8.89) centre (88.9, 6.35) ccw
  line L627 (88.9, 56.896) -> (88.9, 57.404)
  arc A254 (89.5414, 57.15) -> (88.2587, 57.15) centre (88.9, 57.15) ccw
  arc A255 (88.2587, 57.15) -> (89.5414, 57.15) centre (88.9, 57.15) ccw